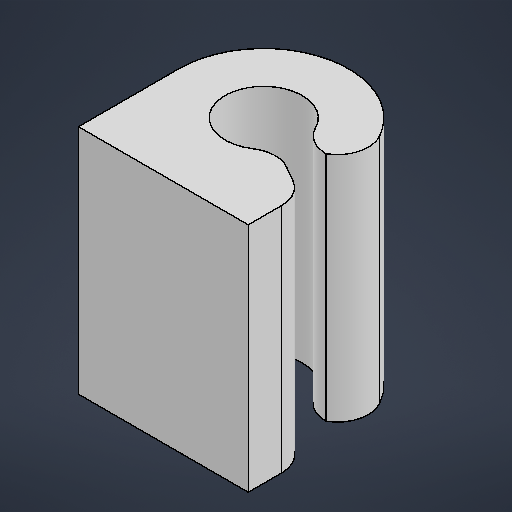
# Autodesk Inventor part: Cable Clip
Saved by Autodesk Inventor 2026.1 (Build 301233000, 233)
## iProperties
Created: 2025-08-27
Part Number: Cable Clip
Material: Generic
Document SubType Name: Modeling
Designer: Joshua Eah
Mass: 1.35176 g
Surface Area: 10.3571 cm^2
Volume: 1.35176 cm^3
Density: 1 g/cm^3
Appearance: Default
Author: Joshua Eah
Autodesk Inventor part; units mm, degrees
ref_plane "YZ Plane" through (0, 0, 0) normal (1, 0, 0) x (0, 1, 0)
ref_plane "XZ Plane" through (0, 0, 0) normal (0, 1, 0) x (-1, 0, 0)
ref_plane "XY Plane" through (0, 0, 0) normal (0, 0, 1) x (1, 0, 0)
sketch "Sketch1" plane through (0, 0, 0) normal (0, 1, 0) x (-1, 0, 0)
  circle A0 centre (0, 0) radius 2.5
  circle A1 centre (0, 0) radius 5.5
  line L0 (5.5, 5.5) -> (-5.5, 5.5)
  line L1 (-5.5, 5.5) -> (-5.5, 6.5)
  line L2 (-5.5, 6.5) -> (5.5, 6.5)
  line L3 (5.5, 6.5) -> (5.5, 5.5)
  line L4 (0, -7.9) -> (0, 8.9) construction
  line L5 (0, 0) -> (-5.5, 3.175426)
  line L6 (0, 0) -> (-5.5, 0)
  line L7 (5.5, 0) -> (5.5, 5.5)
  line L8 (-5.5, 0) -> (-5.5, 5.5)
  point P0 (-2.5, 0)
  point P1 (0, 5.5)
  point P2 (-2.165064, 1.25)
  dimension "d0" = 5
  dimension "d1" = 3
  dimension "d4" = 30
  dimension "d5" = 1
  constraints: 16 end point, 3 point on line, 3 tangent, 2 centre point, 2 coincident, 2 horizontal, 2 parallel, 2 perpendicular, 2 point on circle, 1 collinear, 1 other
  measures "d0" diameter of A0
  measures "d1" radial gap between concentric circles of A1 A0
  measures "d4" angle of L6 L5
  measures "d5" distance between parallel lines of L2 L0
sketch "Sketch1 outline for Extrusion1" plane through (0, 0, 0) normal (0, 1, 0) x (-1, 0, 0)
  line L0 (5.5, 0) -> (5.5, 6.5)
  line L1 (5.5, 6.5) -> (-5.5, 6.5)
  line L2 (-5.5, 6.5) -> (-5.5, 3.175426)
  line L3 (-5.5, 3.175426) -> (-2.165064, 1.25)
  arc A0 (-2.165064, 1.25) -> (-2.5, 0) centre (0, 0) cw
  line L4 (-2.5, 0) -> (-5.5, 0)
  arc A1 (-5.5, 0) -> (5.5, 0) centre (0, 0) ccw
extrude "Extrusion1" add sketch "Sketch1 outline for Extrusion1" along normal blind 15
fillet "Fillet1" radius 2 4 edges at (5.5, 7.5, 3.1754) (2.1651, 7.5, 1.25) (2.5, 7.5, 0) (5.5, 7.5, 0)
body "Solid1"
